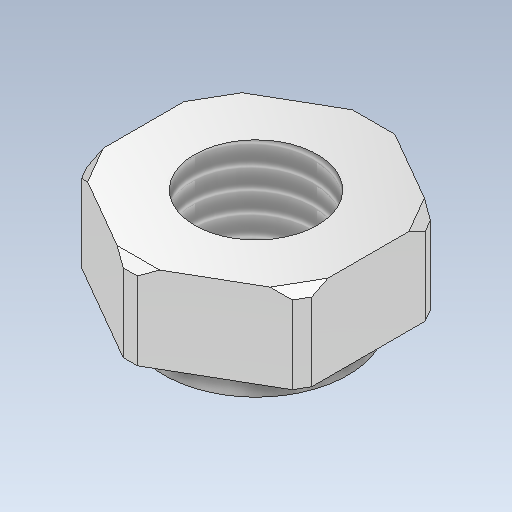
# Autodesk Inventor part: S3-07-3W
Saved by Autodesk Inventor 2020 (Build 240168000, 168)
## iProperties
Created: 2021-09-02
Part Number: S3-07-3W
Material: ステンレス鋼 AISI 304
Document SubType Name: Modeling
Designer: naoki
Density: 8 g/cm^3
Appearance: クロム - サテン
Mass: 0.368542 g
Surface Area: 1.13119 cm^2
Volume: 0.0460677 cm^3
Author: naoki
Autodesk Inventor part; units mm, degrees
ref_plane "YZ Plane" through (0, 0, 0) normal (1, 0, 0) x (0, 1, 0)
ref_plane "XZ Plane" through (0, 0, 0) normal (0, 1, 0) x (-1, 0, 0)
ref_plane "XY Plane" through (0, 0, 0) normal (0, 0, 1) x (1, 0, 0)
sketch "スケッチ2" plane through (0, 0, 0) normal (0, 1, 0) x (-1, 0, 0)
  circle A0 centre (0, 0) radius 1.5
  circle A1 centre (0, 0) radius 2.25
  circle A2 centre (0, 0) radius 2.75
  line L0 (2.75, 2.75) -> (-2.75, -2.75) construction
  line L1 (1.0066, 4.2082) -> (1.0066, -4.7182) construction
  line L2 (3.3819, 0) -> (-4.1959, 0) construction
  line L3 (-2.75, -1.5877) -> (0, -3.1754)
  line L4 (-2.1903, -1.9109) -> (0.8771, -1.9109) construction
  line L5 (-2.75, 0) -> (-2.75, -1.5877)
  line L6 (0, 3.6036) -> (0, -4.7182) construction
  line L7 (-2.75, 1.5877) -> (0, 3.1754)
  line L8 (-2.75, 0) -> (-2.75, 1.5877)
  line L9 (2.75, -1.5877) -> (0, -3.1754)
  line L10 (2.75, 0) -> (2.75, -1.5877)
  line L11 (2.75, 1.5877) -> (0, 3.1754)
  line L12 (2.75, 0) -> (2.75, 1.5877)
  dimension "d8" = 5.5
  dimension "d6" = 3
  dimension "d7" = 4.5
  dimension "d12" = 30
  constraints: 26 end point, 5 symmetric about line, 4 vertical, 3 coincident, 3 point on line, 2 centre point, 2 horizontal, 1 horizontal alignment, 1 midpoint, 1 perpendicular, 4 other
  measures "d6" diameter of A0
  measures "d7" diameter of A1
  measures "d12" angle of L3 L4
extrude "押し出し1" add sketch "スケッチ2" against normal blind 0.7 contours A1
extrude "押し出し2" add sketch "スケッチ2" along normal blind 2.1 contours A1 | A2 | L10 L9 A2 | A2 L11 L12 | A2 L7 L11 | L9 L3 A2 | A2 L8 L7 | L3 L5 A2
chamfer "面取り1" distance 0.2 angle 45 6 edges at (2.75, 1.05, -1.5877) (0, 1.05, -3.1754) (-2.75, 1.05, -1.5877) (-2.75, 1.05, 1.5877) (0, 1.05, 3.1754) (2.75, 1.05, 1.5877)
chamfer "面取り2" distance 0.2 angle 45 6 edges at (2.6634, 2.1, -1.5377) (0, 2.1, -3.0754) (-2.6634, 2.1, -1.5377) (-2.6634, 2.1, 1.5377) (0, 2.1, 3.0754) (2.6634, 2.1, 1.5377)
thread "ねじ1" size "M3x0.5" class "6H" standard "ANSI Metric M Profile" full length
